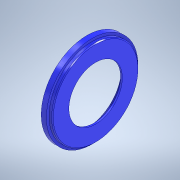
# Autodesk Inventor part: Крышка правая
Saved by Autodesk Inventor 2021 (Build 250183000, 183)
## iProperties
Created: 2023-04-24
Part Number: Крышка правая
Material: Сталь, углеродистая
Document SubType Name: Modeling
Designer: gdevc
Density: 7.85 g/cm^3
Appearance: Синий — малярная краска — глянцевая
Author: gdevc
Autodesk Inventor part; units mm, degrees
ref_plane "YZ Plane" through (0, 0, 0) normal (1, 0, 0) x (0, 1, 0)
ref_plane "XZ Plane" through (0, 0, 0) normal (0, 1, 0) x (-1, 0, 0)
ref_plane "XY Plane" through (0, 0, 0) normal (0, 0, 1) x (1, 0, 0)
sketch "Эскиз1" plane through (0, 0, 0) normal (0, 0, 1) x (1, 0, 0)
  line L0 (0, 0) -> (29.4445, 0)
  line L1 (0, 47.5) -> (3, 47.5)
  line L2 (0, 47.5) -> (0, 44.5)
  line L3 (0, 44.5) -> (3, 44.5)
  line L4 (3, 47.5) -> (3, 53)
  line L5 (3, 53) -> (9, 53)
  line L6 (9, 53) -> (9, 50)
  line L7 (9, 50) -> (13, 50)
  line L8 (13, 50) -> (13, 37.2933)
  line L9 (13, 37.2933) -> (13, 31)
  line L10 (13, 31) -> (11, 31)
  line L11 (11, 31) -> (11, 40)
  line L12 (11, 40) -> (3, 40)
  line L13 (3, 40) -> (3, 44.5)
  dimension "d2" = 62
  dimension "d3" = 100
  dimension "d4" = 3
  dimension "d5" = 6
  dimension "d6" = 89
  dimension "d7" = 80
  dimension "d8" = 8
  dimension "d9" = 0
  dimension "d10" = 13
  dimension "d15" = 3
  dimension "d16" = 3
  constraints: 28 end point, 8 perpendicular, 3 vertical, 2 horizontal, 1 point on line
  measures "d2" diameter of L10 L0
  measures "d3" diameter of L7 L0
  measures "d4" distance between parallel lines of L7 L5
  measures "d5" distance of L4.end L5.end
  measures "d6" diameter of L3 L0
  measures "d7" diameter of L12 L0
  measures "d8" distance of L11.end L12.end
  measures "d9" distance between parallel lines of L4 L13
  measures "d10" distance between parallel lines of L9 L2
  measures "d15" distance between parallel lines of L3 L1
  measures "d16" distance of L1.start L1.end
revolve "Вращение1" add sketch "Эскиз1" angle 360 about axis through (0, 0, 0) along (1, 0, 0)
chamfer "Фаска1" distance 1 angle 45 1 edges at (13, -50, 0)
